Acrylic Support Panels (Autodesk Fusion 360 design; units mm, degrees)
Autodesk Fusion 360 part; units mm, degrees
sketch "Sketch1" plane through (0, 0, 0) normal (1, 0, 0) x (0, 1, 0)
  circle A0 centre (0, 0) radius 2.5
  circle A1 centre (17.3205, 10) radius 2.5
  circle A2 centre (0, 0) radius 5
  circle A3 centre (17.3205, 10) radius 5
  line L0 (-2.5, 4.3301) -> (14.8205, 14.3301)
  line L1 (0, 0) -> (33.5038, 19.3434) construction
  line L2 (0, 0) -> (38.6869, 0) construction
  circle A4 centre (-100, -17.5) radius 7.5
  line L3 (-100, -25) -> (150, -25) construction
  circle A5 centre (-75.588, 163.3599) radius 175
  line L4 (21.6506, 12.5) -> (43.3013, -25)
  line L5 (-100, -25) -> (43.3013, -25)
  circle A6 centre (-100, -17.5) radius 2.5
  line L6 (-100, -17.5) -> (-50, -17.5) construction
  circle A7 centre (-50, -17.5) radius 2.5
  line L7 (-50, -17.5) -> (0, -17.5) construction
  circle A8 centre (0, -17.5) radius 2.5
  dimension "d1" = 5
  dimension "d2" = 5
  dimension "d5" = 10
  dimension "d6" = 30
  dimension "d7" = 15
  dimension "d8" = 100
  dimension "d12" = 25
  dimension "d16" = 20
  dimension "d19" = 350
  dimension "d20" = 5
  dimension "d21" = 5
  dimension "d22" = 50
  dimension "d23" = 50
  dimension "d24" = 5
  constraint coincident A0.centre A2.centre
  constraint concentric A0 A2
  constraint concentric A1 A3
  constraint equal A2 A3
  constraint coincident A2 L0.start
  constraint coincident A3 L0.end
  constraint tangent A3 L0
  constraint tangent A2 L0
  constraint horizontal L2
  constraint coincident A1.centre L1
  constraint horizontal L3
  constraint tangent A4 L3
  constraint tangent A2 A5
  constraint tangent A4 A5
  constraint coincident A3 L4.start
  constraint coincident L1 L4.start
  constraint coincident L3 L4.end
  constraint tangent A3 L4
  constraint coincident A4 L3.start
  constraint tangent A4 L5
  constraint concentric A4 A6
  constraint coincident A4.centre A6.centre
  constraint parallel L5 L6
  constraint coincident L6.end A7.centre
  constraint parallel L6 L7
  constraint coincident L7.end A8.centre
  measures "d1" diameter of A0
  measures "d2" diameter of A1
  measures "d5" diameter of A3
  measures "d6" angle of L1 L2
  measures "d7" diameter of A4
  measures "d8" horizontal distance of A0.centre A4.centre
  measures "d12" distance of A0.centre L3
  measures "d16" distance of A1.centre A0.centre
  measures "d19" diameter of A5
  measures "d20" diameter of A6
  measures "d21" diameter of A7
  measures "d22" distance of A4.centre L6.end
  measures "d23" distance of L6.end L7.end
  measures "d24" diameter of A8
extrude "Extrude1" add sketch "Sketch1" along normal blind 3 contours A2 | A2 L0 A5 | A2 A3 L0 A4 A5 L4 L5 | A3 L0 A5 | A3 A5 | A3 A5 | A4 picked at (4.7327, 8.1697)
fillet "Fillet1" radius 5 1 edges at (1.5, 43.3013, -25)
sketch "Sketch2" plane through (0, 0, 0) normal (1, 0, 0) x (0, 1, 0)
  arc A0 (34.641, -25) -> (38.9711, -17.5) centre (34.641, -20) ccw construction
  line L0 (34.641, -25) -> (-100, -25) construction
  arc A1 (-98.9968, -10.0674) -> (-100, -25) centre (-100, -17.5) ccw construction
  arc A2 (-98.9968, -10.0674) -> (-2.3031, 4.4438) centre (-75.588, 163.3599) ccw construction
  line L1 (-2.3031, 4.4438) -> (14.8205, 14.3301) construction
  arc A3 (21.6506, 12.5) -> (14.8205, 14.3301) centre (17.3205, 10) ccw construction
  line L2 (21.6506, 12.5) -> (38.9711, -17.5) construction
  circle A4 centre (-100, -17.5) radius 2.5 construction
  circle A5 centre (-50, -17.5) radius 2.5 construction
  circle A6 centre (0, -17.5) radius 2.5 construction
  circle A7 centre (17.3205, 10) radius 2.5 construction
  circle A8 centre (0, 0) radius 2.5 construction
  line L3 (39.641, 15) -> (-107.5, 15) construction
  line L4 (-107.5, 15) -> (-107.5, -25) construction
  line L5 (-107.5, -25) -> (39.641, -25) construction
  line L6 (39.641, -25) -> (39.641, 15) construction
  constraint horizontal L3
  constraint vertical L4
  constraint horizontal L5
  constraint vertical L6
  constraint tangent A0 L6
  constraint tangent A1 L4
  constraint tangent A3 L3
  constraint tangent A0 L5
